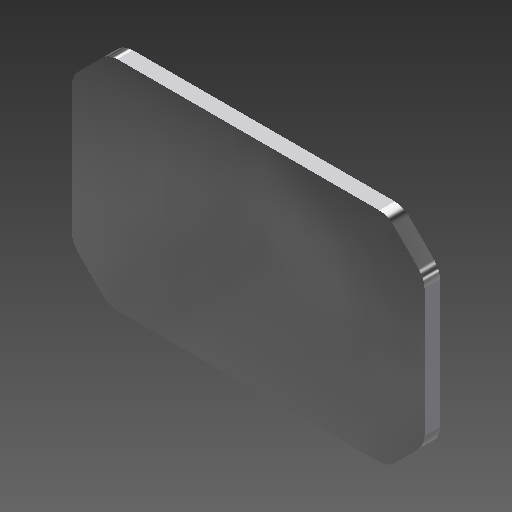
# Autodesk Inventor part: 3d_DAA - Enclosure Glass
Saved by Autodesk Inventor 2018 (Build 220112000, 112)
## iProperties
Category: 0
Created: 2024-05-15
Part Number: 3d_DAA - Enclosure Glass
Material: Genérico
Document SubType Name: Modeling
Designer: cda1
Density: 1 g/cm^3
Appearance: Cromo - Pulido
Manufacturer-1: {"Link": "", "Name": "Knight Optical (UK) Ltd", "PartNumber": "3d_DAA - Enclosure Glass", "partner_id": false}
Manufacturer-2: {"Link": "", "Name": "", "PartNumber": "", "partner_id": false}
Manufacturer-3: {"Link": "", "Name": "", "PartNumber": "", "partner_id": false}
Manufacturer-4: {"Link": "", "Name": "", "PartNumber": "", "partner_id": false}
Manufacturer-5: {"Link": "", "Name": "", "PartNumber": "", "partner_id": false}
Provider-1: {"Link": "", "Name": "", "PartNumber": "", "partner_id": false}
Provider-2: {"Link": "", "Name": "", "PartNumber": "", "partner_id": false}
Provider-3: {"Link": "", "Name": "", "PartNumber": "", "partner_id": false}
Provider-4: {"Link": "", "Name": "", "PartNumber": "", "partner_id": false}
Provider-5: {"Link": "", "Name": "", "PartNumber": "", "partner_id": false}
odoo_id: 17984
odoo_internal_code: P010349
odoo_model: product.product
odoo_x2o_application_version: 12.0.4.10
odoo_d2o_version: 12.0.1.4.34
Author: cda1
Autodesk Inventor part; units mm, degrees
ref_plane "YZ Plane" through (0, 0, 0) normal (1, 0, 0) x (0, 1, 0)
ref_plane "XZ Plane" through (0, 0, 0) normal (0, 1, 0) x (-1, 0, 0)
ref_plane "XY Plane" through (0, 0, 0) normal (0, 0, 1) x (1, 0, 0)
sketch "Boceto1" plane through (0, 0, 0) normal (0, 0, 1) x (1, 0, 0)
  line L0 (3, 0) -> (67, 0)
  line L1 (70, 3) -> (70, 41)
  line L2 (67, 44) -> (3, 44)
  line L3 (0, 41) -> (0, 3)
  arc A0 (3, 44) -> (0, 41) centre (3, 41) ccw
  arc A1 (0, 3) -> (3, 0) centre (3, 3) ccw
  arc A2 (67, 0) -> (70, 3) centre (67, 3) ccw
  arc A3 (70, 41) -> (67, 44) centre (67, 41) ccw
  point P0 (0, 0)
  point P1 (70, 44)
  point P2 (70, 0)
  point P3 (0, 44)
  dimension "d0" = 70
  dimension "d1" = 44
  dimension "d2" = 3
  constraints: 8 end point, 8 point on circle, 8 point on line, 8 tangent, 4 centre point, 3 equal radius, 2 parallel, 1 horizontal, 1 perpendicular
  measures "d0" distance of point (0, 44) point (70, 44)
  measures "d1" distance of point (70, 44) point (70, 0)
  measures "d2" radius of A0
extrude "Extrusión1" add sketch "Boceto1" along normal blind 3
sketch "Boceto2" plane through (0, 0, 3) normal (0, 0, 1) x (1, 0, 0)
  line L0 (0, 41) -> (0, 3) projected
  arc A0 (0, 3) -> (3, 0) centre (3, 3) ccw projected
  line L1 (3, 0) -> (67, 0) projected
  arc A1 (67, 0) -> (70, 3) centre (67, 3) ccw projected
  line L2 (70, 3) -> (70, 41) projected
  arc A2 (70, 41) -> (67, 44) centre (67, 41) ccw projected
  line L3 (67, 44) -> (3, 44) projected
  arc A3 (3, 44) -> (0, 41) centre (3, 41) ccw projected
  line L4 (3, 43) -> (67, 43)
  arc A4 (69, 41) -> (67, 43) centre (67, 41) ccw
  line L5 (69, 41) -> (69, 3)
  arc A5 (67, 1) -> (69, 3) centre (67, 3) ccw
  line L6 (67, 1) -> (3, 1)
  arc A6 (1, 3) -> (3, 1) centre (3, 3) ccw
  line L7 (1, 3) -> (1, 41)
  arc A7 (3, 43) -> (1, 41) centre (3, 41) ccw
  point P0 (0, 0)
  dimension "d5" = 1
  constraints: 8 end point, 8 point on circle, 4 centre point, 7 other
  measures "d5" distance between parallel lines of L3 L4
extrude "Extrusión2" cut sketch "Boceto2" against normal through all
sketch "Boceto5" plane through (0, 0, 3) normal (0, 0, 1) x (1, 0, 0)
  arc A0 (3, 43) -> (1, 41) centre (3, 41) ccw projected
  line L0 (1, 41) -> (1, 3) projected
  arc A1 (1, 3) -> (3, 1) centre (3, 3) ccw projected
  line L1 (3, 1) -> (67, 1) projected
  arc A2 (67, 1) -> (69, 3) centre (67, 3) ccw projected
  line L2 (69, 3) -> (69, 41) projected
  arc A3 (69, 41) -> (67, 43) centre (67, 41) ccw projected
  line L3 (67, 43) -> (3, 43) projected
  arc A4 (2.1716, 37.0858) -> (1, 34.2574) centre (5, 34.2574) ccw
  line L4 (1, 34.2574) -> (1, 9.7426)
  arc A5 (1, 9.7426) -> (2.1716, 6.9142) centre (5, 9.7426) ccw
  line L5 (2.1716, 6.9142) -> (6.9142, 2.1716)
  arc A6 (6.9142, 2.1716) -> (9.7426, 1) centre (9.7426, 5) ccw
  line L6 (9.7426, 1) -> (60.2574, 1)
  arc A7 (60.2574, 1) -> (63.0858, 2.1716) centre (60.2574, 5) ccw
  line L7 (63.0858, 2.1716) -> (67.8284, 6.9142)
  arc A8 (67.8284, 6.9142) -> (69, 9.7426) centre (65, 9.7426) ccw
  line L8 (69, 9.7426) -> (69, 34.2574)
  arc A9 (69, 34.2574) -> (67.8284, 37.0858) centre (65, 34.2574) ccw
  line L9 (67.8284, 37.0858) -> (63.0858, 41.8284)
  arc A10 (63.0858, 41.8284) -> (60.2574, 43) centre (60.2574, 39) ccw
  line L10 (60.2574, 43) -> (9.7426, 43)
  arc A11 (9.7426, 43) -> (6.9142, 41.8284) centre (9.7426, 39) ccw
  line L11 (6.9142, 41.8284) -> (2.1716, 37.0858)
  arc A12 (2.8787, 36.3787) -> (2, 34.2574) centre (5, 34.2574) ccw
  line L12 (2, 34.2574) -> (2, 9.7426)
  arc A13 (2, 9.7426) -> (2.8787, 7.6213) centre (5, 9.7426) ccw
  line L13 (2.8787, 7.6213) -> (7.6213, 2.8787)
  arc A14 (7.6213, 2.8787) -> (9.7426, 2) centre (9.7426, 5) ccw
  line L14 (9.7426, 2) -> (60.2574, 2)
  arc A15 (60.2574, 2) -> (62.3787, 2.8787) centre (60.2574, 5) ccw
  line L15 (62.3787, 2.8787) -> (67.1213, 7.6213)
  arc A16 (67.1213, 7.6213) -> (68, 9.7426) centre (65, 9.7426) ccw
  line L16 (68, 9.7426) -> (68, 34.2574)
  arc A17 (68, 34.2574) -> (67.1213, 36.3787) centre (65, 34.2574) ccw
  line L17 (67.1213, 36.3787) -> (62.3787, 41.1213)
  arc A18 (62.3787, 41.1213) -> (60.2574, 42) centre (60.2574, 39) ccw
  line L18 (60.2574, 42) -> (9.7426, 42)
  arc A19 (9.7426, 42) -> (7.6213, 41.1213) centre (9.7426, 39) ccw
  line L19 (7.6213, 41.1213) -> (2.8787, 36.3787)
  point P0 (0, 0)
  dimension "d0" = 70
  dimension "d1" = 44
  dimension "d2" = 3
  dimension "d23" = 1
  dimension "d24" = 4
  dimension "d25" = 8.7426
  dimension "d26" = 4
  dimension "d27" = 8.7426
  dimension "d28" = 4
  dimension "d29" = 4
  dimension "d30" = 8.7426
  dimension "d31" = 4
  dimension "d32" = 8.7426
  dimension "d33" = 4
  dimension "d34" = 4
  dimension "d35" = 8.7426
  dimension "d36" = 8.7426
  dimension "d37" = 4
  dimension "d38" = 8.7426
  dimension "d39" = 8.7426
  dimension "d40" = 4
  dimension "d41" = 4
  dimension "d42" = 4
  dimension "d43" = 1
  dimension "d44" = 1
  dimension "d45" = 4
  dimension "d46" = 4
  dimension "d47" = 1
  dimension "d48" = 4
  dimension "d49" = 4
  dimension "d50" = 4
  dimension "d51" = 45
  dimension "d52" = 45
  dimension "d53" = 45
  dimension "d54" = 45
  dimension "d55" = 90
  dimension "d56" = 90
  constraints: 32 end point, 32 point on circle, 16 centre point, 15 other
  measures "d23" distance between parallel lines of L11 L19
  measures "d24" radius of A8
  measures "d25" distance from line of L1 A8.centre
  measures "d26" distance from line of L2 A8.centre
  measures "d27" distance from line of L2 A7.centre
  measures "d28" distance from line of L1 A7.centre
  measures "d29" distance from line of L3 A10.centre
  measures "d30" distance from line of A10.centre L2
  measures "d31" distance from line of L2 A9.centre
  measures "d32" distance from line of L3 A9.centre
  measures "d33" distance from line of L0 A5.centre
  measures "d34" distance from line of L1 A6.centre
  measures "d35" distance from line of L1 A5.centre
  measures "d36" distance from line of L0 A6.centre
  measures "d37" distance from line of L0 A4.centre
  measures "d38" distance from line of L3 A4.centre
  measures "d39" distance from line of L0 A11.centre
  measures "d40" distance from line of L3 A11.centre
  measures "d41" radius of A11
  measures "d42" radius of A4
  measures "d43" distance between parallel lines of L0 L12
  measures "d44" distance between parallel lines of L1 L14
  measures "d45" radius of A9
  measures "d46" radius of A10
  measures "d47" distance from line of L2.end L16
  measures "d48" radius of A7
  measures "d49" radius of A6
  measures "d50" radius of A5
  measures "d51" angle of L0 L11
  measures "d52" angle of L0 L5
  measures "d53" angle of L2 L7
  measures "d54" angle of L2 L9
  measures "d55" angle of L18 L0
  measures "d56" angle of L3 L16
extrude "Extrusión4" cut sketch "Boceto5" against normal through all contours L3 A11 L11 A4 L0 A0 | L3 A3 L2 A9 L9 A10 | A5 L5 A6 L1 A1 L0 | L2 A2 L1 A7 L7 A8
